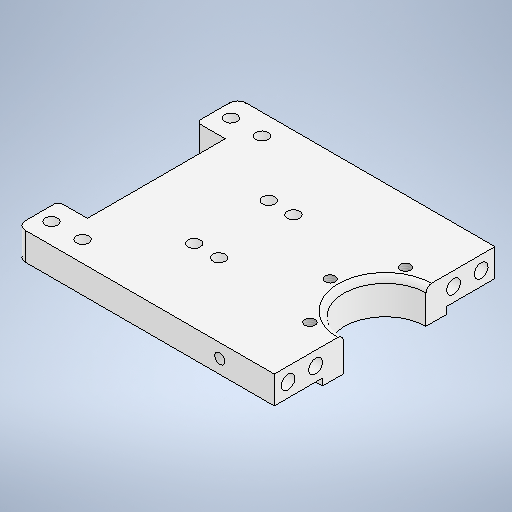
# Autodesk Inventor part: joint4_base
Saved by Autodesk Inventor 2025.3 (Build 293356030, 356C)
## iProperties
Created: 2025-11-08
Part Number: joint4_base
Material: PLA filament
Document SubType Name: Modeling
Designer: MSI
Density: 1.2 g/cm^3
Appearance: 일반
Mass: 75.0376 g
Surface Area: 204.664 cm^2
Volume: 62.5313 cm^3
Author: MSI
Autodesk Inventor part; units mm, degrees
ref_plane "YZ Plane" through (0, 0, 0) normal (1, 0, 0) x (0, 1, 0)
ref_plane "XZ Plane" through (0, 0, 0) normal (0, 1, 0) x (-1, 0, 0)
ref_plane "XY Plane" through (0, 0, 0) normal (0, 0, 1) x (1, 0, 0)
sketch "스케치1" plane through (0, 0, 0) normal (0, 1, 0) x (-1, 0, 0)
  line L0 (93.5, 40) -> (-93.5, 40)
  line L1 (-93.5, 40) -> (-93.5, -40)
  line L2 (-93.5, -40) -> (93.5, -40)
  line L3 (93.5, -40) -> (93.5, 40)
  line L4 (93.5, 40) -> (-93.5, -40) construction
  line L5 (-93.5, 40) -> (93.5, -40) construction
  point P0 (0, 0)
  dimension "d0" = 187
  dimension "d1" = 80
  constraints: 12 end point, 2 midpoint, 2 parallel, 1 horizontal, 1 perpendicular
  measures "d0" distance of L0.start L0.end
  measures "d1" distance of L0.end L1.end
extrude "돌출1" add sketch "스케치1" along normal mid plane 10
sketch "스케치2" plane through (0, -5, 0) normal (0, -1, 0) x (1, 0, 0)
  line L0 (25.9808, 0) -> (12.9904, -22.5)
  line L1 (12.9904, -22.5) -> (-12.9904, -22.5)
  line L2 (-12.9904, -22.5) -> (-25.9808, 0)
  line L3 (-25.9808, 0) -> (-12.9904, 22.5)
  line L4 (-12.9904, 22.5) -> (12.9904, 22.5)
  line L5 (12.9904, 22.5) -> (25.9808, 0)
  point P0 (0, 0)
  point P1 (0, 0)
  dimension "d4" = 45
  constraints: 12 end point, 1 coincident, 1 horizontal, 13 other
  measures "d4" distance between parallel lines of L1 L4
extrude "돌출2" add sketch "스케치2" along normal blind 2.5
sketch "스케치3" plane through (0, 5, 0) normal (0, 1, 0) x (1, 0, 0)
  line L0 (-93.5, -40) -> (-93.5, 40) projected
  line L1 (-93.5, 25) -> (-83, 25)
  line L2 (-83, 25) -> (-83, -25)
  line L3 (-83, -25) -> (-93.5, -25)
  line L4 (-93.5, -25) -> (-93.5, 25)
  line L5 (93.5, 40) -> (-93.5, 40) projected
  point P0 (0, 0)
  point P1 (-83, 0)
  point P2 (-93.5, -25)
  dimension "d7" = 15
  dimension "d8" = 10.5
  constraints: 8 end point, 2 parallel, 1 horizontal, 1 horizontal alignment, 1 midpoint, 1 perpendicular, 1 point on line
  measures "d7" distance between parallel lines of L5 L1
  measures "d8" distance of L2.end L3.end
extrude "돌출3" cut sketch "스케치3" against normal through all
mirror "미러1" about plane through (0, 0, 0) normal (1, 0, 0) of "돌출3"
sketch "스케치4" plane through (0, 5, 0) normal (0, 1, 0) x (1, 0, 0)
  point P0 (0, 0)
hole "구멍1" at (0, 5, 0) direction (0, -1, 0) diameter 30 end through all
sketch "스케치5" plane through (0, -5, 0) normal (0, -1, 0) x (1, 0, 0)
  line L0 (58.779, 16.5) -> (43.779, 16.5) construction
  line L1 (43.779, 16.5) -> (43.779, -16.5) construction
  line L2 (43.779, -16.5) -> (58.779, -16.5) construction
  line L3 (58.779, -16.5) -> (58.779, 16.5) construction
  circle A0 centre (0, 0) radius 15 projected
  line L4 (55.779, -13.5) -> (46.779, -13.5)
  line L5 (46.779, -13.5) -> (46.779, 13.5)
  line L6 (46.779, 13.5) -> (55.779, 13.5)
  line L7 (55.779, 13.5) -> (55.779, -13.5)
  line L8 (-12.9904, 22.5) -> (12.9904, 22.5) projected
  line L9 (0, 22.5) -> (0, -22.4206)
  line L10 (-58.779, 16.5) -> (-43.779, 16.5) construction
  line L11 (-43.779, 16.5) -> (-43.779, -16.5) construction
  line L12 (-43.779, -16.5) -> (-58.779, -16.5) construction
  line L13 (-58.779, -16.5) -> (-58.779, 16.5) construction
  line L14 (-55.779, -13.5) -> (-46.779, -13.5)
  line L15 (-46.779, -13.5) -> (-46.779, 13.5)
  line L16 (-46.779, 13.5) -> (-55.779, 13.5)
  line L17 (-55.779, 13.5) -> (-55.779, -13.5)
  point P0 (43.779, 0)
  point P1 (-43.779, 0)
  dimension "d18" = 43.779
  dimension "d19" = 15
  dimension "d20" = 33
  dimension "d21" = 3
  constraints: 34 end point, 13 symmetric about line, 8 coincident, 4 parallel, 2 midpoint, 2 perpendicular, 1 horizontal, 1 horizontal alignment, 1 vertical, 3 other
  measures "d18" distance from line of L1 A0.centre
  measures "d19" distance of L0.start L0.end
  measures "d20" distance of L2.end L0.start
  measures "d21" distance between parallel lines of L2 L4
hole "구멍2" at (55.779, -5, 13.5) at (46.779, -5, 13.5) at (46.779, -5, -13.5) at (55.779, -5, -13.5) at (-55.779, -5, -13.5) at (-46.779, -5, -13.5) at (-46.779, -5, 13.5) at (-55.779, -5, 13.5) direction (0, 1, 0) diameter 4.5 end through all counterbore diameter 8 counterbore depth 4.4 clearance for "Socket Head Cap Screw ISO 4762" size "M4" standard "ISO"
sketch "스케치6" plane through (0, -7.5, 0) normal (0, -1, 0) x (1, 0, 0)
  line L0 (0, 0) -> (-20, 0)
  dimension "d30" = 20
  constraints: 2 end point, 1 horizontal
  measures "d30" distance of L0.start L0.end
hole "구멍3" at (-20, -7.5, 0) direction (0, 1, 0) diameter 3.6881 end through all thread size "M4.5x0.75" class "6H" standard "ISO Metric profile"
pattern_circular "원형 패턴1" count 6 over 360 about axis through (0, -198.7775, 0) along (0, 1, 0) of "구멍3"
sketch "스케치7" plane through (83, -5, -25) normal (1, 0, 0) x (0, 0, -1)
  line L0 (-43.375, 5) -> (-6.625, 5)
  point P0 (-25, 5)
  point P1 (-25, 5)
  point P2 (-31.125, 5)
  point P3 (-18.875, 5)
  dimension "d41" = 12.25
  dimension "d42" = 12.25
  dimension "d43" = 36.75
  constraints: 3 coincident, 2 end point, 2 point on line, 1 horizontal, 1 midpoint
  measures "d41" distance of point (-31.125, 5) L0.start
  measures "d42" distance of point (-18.875, 5) point (-6.625, 5)
  measures "d43" distance of L0.start L0.end
hole "구멍4" at (83, 0, 18.375) at (83, 0, 6.125) at (83, 0, -18.375) at (83, 0, -6.125) direction (-1, 0, 0) diameter 3.6881 depth 13 tip angle 118 thread size "M4.5x0.75" class "6H" standard "ISO Metric profile"
sketch "스케치8" plane through (0, -5, 0) normal (0, -1, 0) x (1, 0, 0)
  line L0 (88.5, 32.5) -> (77.25, 32.5)
  line L1 (77.25, 32.5) -> (77.25, -32.5)
  line L2 (77.25, -32.5) -> (88.5, -32.5)
  line L3 (88.5, -32.5) -> (88.5, 32.5)
  line L4 (93.5, 25) -> (93.5, 40) projected
  line L5 (93.5, -40) -> (93.5, -25) projected
  point P0 (0, 0)
  point P1 (93.5, 32.5)
  point P2 (93.5, -32.5)
  dimension "d51" = 11.25
  dimension "d84" = 5
  constraints: 8 end point, 4 coincident, 2 midpoint, 2 parallel, 2 point on line, 1 horizontal, 1 perpendicular
  measures "d51" distance of L0.start L0.end
  measures "d84" distance between parallel lines of L4 L3
hole "구멍5" at (88.5, -5, 32.5) at (77.25, -5, 32.5) at (77.25, -5, -32.5) at (88.5, -5, -32.5) direction (0, 1, 0) diameter 4.5 end through all counterbore diameter 8 counterbore depth 4.4 clearance for "Socket Head Cap Screw ISO 4762" size "M4" standard "ISO"
mirror "미러2" about plane through (0, 0, 0) normal (1, 0, 0) of "구멍4", "구멍5"
sketch "스케치11" plane through (-93.5, 5, 40) normal (0, 0, 1) x (1, 0, 0)
  line L0 (73.5, -5) -> (113.5, -5) construction
  point P0 (93.5, -5)
  point P1 (93.5, -5)
  dimension "d76" = 40
  constraints: 3 coincident, 2 end point, 1 horizontal, 1 midpoint
  measures "d76" distance of L0.start L0.end
hole "구멍7" at (-20, 0, 40) at (20, 0, 40) direction (0, 0, -1) diameter 3.6881 depth 13 tip angle 118 thread size "M4.5x0.75" class "6H" standard "ISO Metric profile"
mirror "미러3" about plane through (0, 0, 0) normal (0, 0, 1) of "구멍7"
fillet "모깎기1" radius 3 10 edges at (-25.9808, -6.25, 0) (-12.9904, -6.25, 22.5) (12.9904, -6.25, 22.5) (12.9904, -6.25, -22.5) (25.9808, -6.25, 0) (-12.9904, -6.25, -22.5) (-93.5, 0, 40) (-93.5, 0, -40) (93.5, 0, 40) (93.5, 0, -40)
fillet "모깎기2" radius 2 1 edges at (0, 5, -15)
chamfer "모따기1" distance 1 angle 45 4 edges at (93.5, 0, -25) (93.5, 0, 25) (-93.5, 0, -25) (-93.5, 0, 25)
sketch "스케치9" plane through (0, 0, 0) normal (0, 0, 1) x (1, 0, 0)
  line L0 (-0.25, -52.7225) -> (-108.7982, -52.7225)
  line L1 (-108.7982, -52.7225) -> (-108.7982, 52.7225)
  line L2 (-108.7982, 52.7225) -> (-0.25, 52.7225)
  line L3 (-0.25, 52.7225) -> (-0.25, -52.7225)
  point P0 (0, 0)
  point P1 (-0.25, 0)
  dimension "d65" = 0.25
  constraints: 8 end point, 2 parallel, 1 horizontal, 1 horizontal alignment, 1 midpoint, 1 perpendicular
  measures "d65" distance from line of point (0, 0) L3
extrude "돌출4" cut sketch "스케치9" along normal through all both and the other way through all keep common part
sketch "스케치10" plane through (-0.25, 0, 0.0063) normal (1, 0, 0) x (0, 1, 0)
  line L0 (0, 34.9937) -> (0, -35.0063) construction
  point P0 (0, -0.0063)
  point P1 (0, -0.0063)
  point P2 (0, -25.0063)
  point P3 (0, 24.9937)
  dimension "d66" = 70
  dimension "d67" = 10
  dimension "d68" = 10
  constraints: 3 coincident, 2 end point, 2 point on line, 1 midpoint, 1 vertical
  measures "d66" distance of L0.start L0.end
  measures "d67" distance of point (0, 24.994) L0.start
  measures "d68" distance of point (0, -35.006) point (0, -25.006)
hole "구멍6" at (-0.25, 0, 35) at (-0.25, 0, -35) at (-0.25, 0, -25) at (-0.25, 0, 25) direction (-1, 0, 0) diameter 5 depth 10 tip angle 118
equation "\"d42\" = d41"
equation "\"d43\" = 3 * d41"
equation "\"d68\" = d67"
